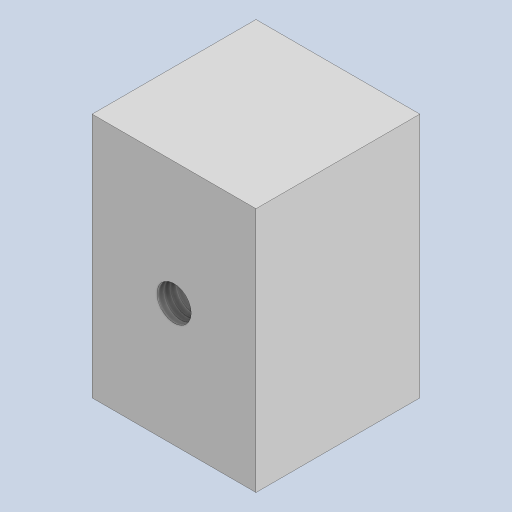
# Autodesk Inventor part: Aluminium block
Saved by Autodesk Inventor 2023.4 (Build 274418000, 418)
## iProperties
Created: 2024-01-11
Part Number: Aluminium block
Material: Generic
Document SubType Name: Modeling
Designer: PalumaCMM
Density: 1 g/cm^3
Appearance: Default
Author: PalumaCMM
Autodesk Inventor part; units mm, degrees
ref_plane "YZ Plane" through (0, 0, 0) normal (1, 0, 0) x (0, 1, 0)
ref_plane "XZ Plane" through (0, 0, 0) normal (0, 1, 0) x (-1, 0, 0)
ref_plane "XY Plane" through (0, 0, 0) normal (0, 0, 1) x (1, 0, 0)
sketch "Sketch1" plane through (0, 0, 0) normal (0, 0, 1) x (1, 0, 0)
  line L0 (0, 0) -> (40, 0)
  line L1 (40, 0) -> (40, 60)
  line L2 (40, 60) -> (0, 60)
  line L3 (0, 60) -> (0, 0)
  dimension "d0" = 40
  dimension "d1" = 60
  constraints: 8 end point, 2 parallel, 1 horizontal, 1 perpendicular
  measures "d0" distance of L2.end L1.end
  measures "d1" distance of L1.end L0.end
extrude "Extrusion1" add sketch "Sketch1" along normal blind 40
sketch "Sketch2" plane through (0, 0, 40) normal (0, 0, 1) x (1, 0, 0)
  circle A0 centre (20, 30) radius 6
  line L0 (0, 0) -> (40, 0) projected
  line L1 (40, 0) -> (40, 60) projected
  point P0 (20, 0)
  dimension "d4" = 12
  dimension "d12" = 30
  dimension "d13" = 20
  constraints: 1 centre point, 1 midpoint
  measures "d4" diameter of A0
  measures "d12" distance of point (20, 0) A0.centre
  measures "d13" distance from line of L1 A0.centre
hole "Hole1" at (20, 30, 40) direction (0, 0, -1) diameter 8.376 end through all thread size "M10x1.5" class "6H" standard "ISO Metric profile"
body "Solid1"
